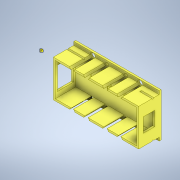
# Autodesk Inventor part: usbHubCaseForTripodClamp
Saved by Autodesk Inventor 2021.2 (Build 252289000, 289)
## iProperties
Created: 2021-02-17
Part Number: usbHubCaseForTripodClamp
Material: PC/ABS Plastic
Document SubType Name: Modeling
Designer: robst
Density: 0.357273 g/cm^3
Appearance: Smooth - Yellow
Author: robst
Autodesk Inventor part; units mm, degrees
ref_plane "YZ Plane" through (0, 0, 0) normal (1, 0, 0) x (0, 1, 0)
ref_plane "XZ Plane" through (0, 0, 0) normal (0, 1, 0) x (-1, 0, 0)
ref_plane "XY Plane" through (0, 0, 0) normal (0, 0, 1) x (1, 0, 0)
sketch "Sketch1" plane through (0, 0, 0) normal (0, 0, 1) x (1, 0, 0)
  line L0 (-57.15, -29.21) -> (57.15, -29.21)
  line L1 (57.15, -29.21) -> (57.15, 29.21)
  line L2 (57.15, 29.21) -> (-57.15, 29.21)
  line L3 (-57.15, 29.21) -> (-57.15, -29.21)
  line L4 (-57.15, -29.21) -> (57.15, 29.21) construction
  line L5 (57.15, -29.21) -> (-57.15, 29.21) construction
  point P0 (0, 0)
  dimension "d0" = 58.42
  dimension "d1" = 114.3
  constraints: 12 end point, 2 midpoint, 2 parallel, 1 horizontal, 1 perpendicular
  measures "d0" distance of L2.end L0.start
  measures "d1" distance of L1.end L2.end
extrude "Extrusion1" add sketch "Sketch1" against normal blind 2.54
sketch "Sketch2" plane through (0, 0, 0) normal (0, 0, 1) x (1, 0, 0)
  line L0 (-57.15, -29.21) -> (-57.15, 29.21) projected
  line L1 (57.15, 29.21) -> (57.15, -29.21) projected
  line L2 (-57.15, 24.765) -> (57.15, 24.765)
  line L3 (57.15, 24.765) -> (57.15, 22.225)
  line L4 (57.15, 22.225) -> (-57.15, 22.225)
  line L5 (-57.15, 22.225) -> (-57.15, 24.765)
  line L6 (-57.15, -24.765) -> (57.15, -24.765)
  line L7 (57.15, -24.765) -> (57.15, -22.225)
  line L8 (57.15, -22.225) -> (-57.15, -22.225)
  line L9 (-57.15, -22.225) -> (-57.15, -24.765)
  point P0 (0, 0)
  point P1 (-57.15, -22.225)
  point P2 (57.15, -24.765)
  dimension "d4" = 2.54
  dimension "d5" = 2.54
  dimension "d6" = 22.225
  dimension "d7" = 22.225
  constraints: 16 end point, 4 parallel, 4 point on line, 2 horizontal, 2 perpendicular
  measures "d4" distance between parallel lines of L4 L2
  measures "d5" distance between parallel lines of L6 L8
  measures "d6" distance from line of L4 point (0, 0)
  measures "d7" distance from line of L8 point (0, 0)
extrude "Extrusion2" add sketch "Sketch2" along normal blind 27.432 contours L0 L8 L1 L6 | L0 L2 L1 L4
sketch "Sketch3" plane through (0, 0, -2.54) normal (0, 0, -1) x (-1, 0, 0)
  line L0 (-12.7, -25.4) -> (12.7, -25.4) construction
  line L1 (12.7, -25.4) -> (12.7, 25.4) construction
  line L2 (12.7, 25.4) -> (-12.7, 25.4) construction
  line L3 (-12.7, 25.4) -> (-12.7, -25.4) construction
  line L4 (-12.7, -25.4) -> (12.7, 25.4) construction
  line L5 (12.7, -25.4) -> (-12.7, 25.4) construction
  point P0 (0, 0)
  dimension "d10" = 25.4
  dimension "d11" = 50.8
  constraints: 12 end point, 4 coincident, 2 midpoint, 2 parallel, 1 horizontal, 1 perpendicular
  measures "d10" distance of L1.end L2.end
  measures "d11" distance of L2.end L0.start
hole "Hole1" at (12.7, 25.4, -2.54) at (-12.7, 25.4, -2.54) at (-12.7, -25.4, -2.54) at (12.7, -25.4, -2.54) direction (0, 0, 1) diameter 3.81 end through all clearance for "Flat Head Machine Screw (82)" size "#6" standard "Ansi Unified Screw Threads"
sketch "Sketch4" plane through (0, 0, 0) normal (0, 0, 1) x (1, 0, 0)
  circle A0 centre (-12.7, 25.4) radius 1.905 projected
  circle A1 centre (-12.7, 25.4) radius 3.81
  circle A2 centre (12.7, 25.4) radius 1.905 projected
  circle A3 centre (12.7, 25.4) radius 3.81
  circle A4 centre (12.7, -25.4) radius 1.905 projected
  circle A5 centre (12.7, -25.4) radius 3.81
  arc A6 (-14.4961, -24.765) -> (-10.9039, -24.765) centre (-12.7, -25.4) ccw projected
  circle A7 centre (-12.7, -25.4) radius 3.81
  point P0 (0, 0)
  dimension "d19" = 7.62
  constraints: 4 centre point, 4 coincident, 3 equal radius
  measures "d19" diameter of A1
extrude "Extrusion3" cut sketch "Sketch4" along normal through all contours A0 | A1 | A2 | A3 | A4 | A5 | A7
sketch "Sketch5" plane through (57.15, -29.21, -2.54) normal (1, 0, 0) x (0, 0, -1)
  line L0 (-29.972, 53.975) -> (-29.972, 51.435) projected
  line L1 (-2.54, 51.435) -> (-2.54, 6.985) projected
  line L2 (-29.972, 51.435) -> (-2.54, 51.435)
  line L3 (-2.54, 51.435) -> (-2.54, 6.985)
  line L4 (-2.54, 6.985) -> (-29.972, 6.985)
  line L5 (-29.972, 6.985) -> (-29.972, 51.435)
  point P0 (-2.54, 29.21)
  constraints: 8 end point, 2 parallel, 1 horizontal, 1 perpendicular
extrude "Extrusion4" add sketch "Sketch5" against normal blind 2.54
sketch "Sketch6" plane through (57.15, -29.21, -2.54) normal (1, 0, 0) x (0, 0, -1)
  line L0 (-2.54, 51.435) -> (-29.972, 51.435) projected
  line L1 (-2.54, 6.985) -> (-2.54, 51.435) projected
  line L2 (-29.972, 6.985) -> (-2.54, 6.985) projected
  line L3 (-29.972, 51.435) -> (-29.972, 53.975) construction
  line L4 (-29.972, 51.435) -> (-2.54, 6.985) construction
  line L5 (-2.54, 51.435) -> (-29.972, 6.985) construction
  line L6 (-23.876, 19.685) -> (-8.636, 19.685)
  line L7 (-8.636, 19.685) -> (-8.636, 38.735)
  line L8 (-8.636, 38.735) -> (-23.876, 38.735)
  line L9 (-23.876, 38.735) -> (-23.876, 19.685)
  line L10 (-23.876, 19.685) -> (-8.636, 38.735) construction
  line L11 (-8.636, 19.685) -> (-23.876, 38.735) construction
  point P0 (-2.54, 29.21)
  point P1 (-16.256, 29.21)
  dimension "d24" = 15.24
  dimension "d25" = 19.05
  constraints: 16 end point, 3 midpoint, 2 parallel, 1 horizontal, 1 perpendicular
  measures "d24" distance of L7.end L8.end
  measures "d25" distance of L6.end L7.end
extrude "Extrusion5" cut sketch "Sketch6" against normal up to surface (2.54 mm away)
sketch "Sketch7" plane through (-57.15, -29.21, -2.54) normal (-1, 0, 0) x (0, 0, 1)
  line L0 (2.54, 51.435) -> (29.972, 51.435) projected
  line L1 (29.972, 6.985) -> (29.972, 51.435) projected
  line L2 (2.54, 6.985) -> (29.972, 6.985) projected
  line L3 (2.54, 51.435) -> (2.54, 6.985) projected
  line L4 (2.54, 6.985) -> (2.54, 51.435) construction
  line L5 (29.972, 6.985) -> (2.54, 6.985) construction
  line L6 (2.54, 51.435) -> (29.972, 6.985) construction
  line L7 (2.54, 51.435) -> (29.972, 51.435) construction
  line L8 (29.972, 51.435) -> (2.54, 6.985) construction
  line L9 (5.461, 13.97) -> (27.051, 13.97)
  line L10 (27.051, 13.97) -> (27.051, 44.45)
  line L11 (27.051, 44.45) -> (5.461, 44.45)
  line L12 (5.461, 44.45) -> (5.461, 13.97)
  line L13 (5.461, 13.97) -> (27.051, 44.45) construction
  line L14 (27.051, 13.97) -> (5.461, 44.45) construction
  point P0 (2.54, 29.21)
  point P1 (16.256, 29.21)
  dimension "d28" = 30.48
  dimension "d29" = 21.59
  constraints: 16 end point, 3 midpoint, 2 parallel, 2 perpendicular
  measures "d28" distance of L11.end L9.start
  measures "d29" distance of L10.end L11.end
extrude "Extrusion6" add sketch "Sketch7" against normal blind 2.54
sketch "Sketch8" plane through (57.15, -29.21, -2.54) normal (1, 0, 0) x (0, 0, -1)
  line L0 (-2.54, 53.975) -> (-29.972, 53.975) projected
  line L1 (-29.972, 53.975) -> (-2.54, 53.975) projected
  line L2 (-12.192, 53.975) -> (-10.922, 52.705)
  line L3 (-10.922, 52.705) -> (-9.652, 53.975)
  line L4 (-9.652, 53.975) -> (-12.192, 53.975)
  line L5 (-29.972, 4.445) -> (-29.972, 53.975) projected
  point P0 (-2.54, 29.21)
  dimension "d32" = 90
  dimension "d33" = 135
  dimension "d34" = 1.27
  dimension "d35" = 19.05
  constraints: 6 end point, 2 point on line, 1 collinear
  measures "d32" angle of L3 L2
  measures "d33" angle of L2 L0
  measures "d34" distance from line of L2.end L0
  measures "d35" distance from line of L2.end L5
extrude "Extrusion7" cut sketch "Sketch8" against normal blind 16.51
mirror "Mirror1" about plane through (0, 0, 0) normal (0, 1, 0) of "Extrusion7"
sketch "Sketch9" plane through (-57.15, -29.21, -2.54) normal (-1, 0, 0) x (0, 0, 1)
  line L0 (9.652, 53.975) -> (10.922, 52.705) projected
  line L1 (10.922, 52.705) -> (12.192, 53.975) projected
  line L2 (2.54, 53.975) -> (29.972, 53.975) projected
  line L3 (12.192, 53.975) -> (10.922, 52.705)
  line L4 (9.652, 53.975) -> (10.922, 52.705) projected
  line L5 (10.922, 52.705) -> (9.652, 53.975)
  line L6 (9.652, 53.975) -> (12.192, 53.975)
  line L7 (2.54, 53.975) -> (29.972, 53.975) projected
  point P0 (2.54, 29.21)
  constraints: 6 end point, 2 collinear
extrude "Extrusion8" cut sketch "Sketch9" against normal blind 27.94
mirror "Mirror2" about plane through (0, 0, 0) normal (0, 1, 0) of "Extrusion8"
sketch "Sketch10" plane through (0, 0, -2.54) normal (0, 0, -1) x (-1, 0, 0)
  line L0 (-31.75, -25.4) -> (31.75, -25.4) construction
  line L1 (31.75, -25.4) -> (31.75, 25.4) construction
  line L2 (31.75, 25.4) -> (-31.75, 25.4) construction
  line L3 (-31.75, 25.4) -> (-31.75, -25.4) construction
  line L4 (-31.75, -25.4) -> (31.75, 25.4) construction
  line L5 (31.75, -25.4) -> (-31.75, 25.4) construction
  point P0 (0, 0)
  dimension "d40" = 63.5
  dimension "d41" = 50.8
  constraints: 12 end point, 4 coincident, 2 midpoint, 2 parallel, 1 horizontal, 1 perpendicular
  measures "d40" distance of L0.start L0.end
  measures "d41" distance of L1.end L0.end
hole "Hole2" at (31.75, 25.4, -2.54) at (-31.75, 25.4, -2.54) at (-31.75, -25.4, -2.54) at (31.75, -25.4, -2.54) direction (0, 0, 1) diameter 6.985 end through all
sketch "Sketch11" plane through (0, 0, 0) normal (0, 0, 1) x (1, 0, 0)
  line L0 (54.61, 9.525) -> (54.61, -9.525) construction
  line L1 (54.61, 0) -> (-54.61, 0) construction
  line L2 (-54.61, 22.225) -> (-54.61, -22.225) construction
  line L3 (-29.5043, -3.81) -> (-30.5171, -3.81)
  line L4 (-30.5171, -3.81) -> (-30.5171, -0.0803)
  line L5 (-30.5171, -0.0803) -> (-34.0245, -0.0803)
  line L6 (-34.0245, -0.0803) -> (-34.0245, -3.81)
  line L7 (-34.0245, -3.81) -> (-35.0372, -3.81)
  line L8 (-35.0372, -3.81) -> (-35.0372, 3.81)
  line L9 (-35.0372, 3.81) -> (-34.0245, 3.81)
  line L10 (-34.0245, 3.81) -> (-34.0245, 0.8213)
  line L11 (-34.0245, 0.8213) -> (-30.5171, 0.8213)
  line L12 (-30.5171, 0.8213) -> (-30.5171, 3.81)
  line L13 (-30.5171, 3.81) -> (-29.5043, 3.81)
  line L14 (-29.5043, 3.81) -> (-29.5043, -3.81)
  spline S0 degree 2 poles (-25.8364, -3.9459) (-26.6638, -3.9459) (-27.8247, -3.6) (-28.3373, -3.353) knots 0 0 0 1 2 2 2
  line L15 (-28.3373, -3.353) -> (-28.3373, -2.081)
  line L16 (-28.3373, -2.081) -> (-28.2632, -2.081)
  spline S1 degree 2 poles (-28.2632, -2.081) (-27.763, -2.5503) (-26.4971, -3.069) (-25.9105, -3.069) knots 0 0 0 1 2 2 2
  spline S2 degree 2 poles (-25.9105, -3.069) (-25.0707, -3.069) (-24.2123, -2.3712) (-24.2123, -1.7969) knots 0 0 0 1 2 2 2
  spline S3 degree 2 poles (-24.2123, -1.7969) (-24.2123, -1.34) (-24.6631, -0.7719) (-25.1509, -0.6299) knots 0 0 0 1 2 2 2
  spline S4 degree 2 poles (-25.1509, -0.6299) (-25.5029, -0.5311) (-26.0895, -0.3952) (-26.528, -0.2841) knots 0 0 0 1 2 2 2
  spline S5 degree 2 poles (-26.528, -0.2841) (-26.9232, -0.1791) (-27.5469, 0.1359) (-27.7877, 0.389) knots 0 0 0 1 2 2 2
  spline S6 degree 2 poles (-27.7877, 0.389) (-28.0223, 0.6422) (-28.2817, 1.3215) (-28.2817, 1.7661) knots 0 0 0 1 2 2 2
  spline S7 degree 2 poles (-28.2817, 1.7661) (-28.2817, 2.6923) (-26.8367, 3.9459) (-25.719, 3.9459) knots 0 0 0 1 2 2 2
  spline S8 degree 2 poles (-25.719, 3.9459) (-25.0768, 3.9459) (-23.9406, 3.6927) (-23.4528, 3.4518) knots 0 0 0 1 2 2 2
  line L17 (-23.4528, 3.4518) -> (-23.4528, 2.2415)
  line L18 (-23.4528, 2.2415) -> (-23.5269, 2.2415)
  spline S9 degree 2 poles (-23.5269, 2.2415) (-23.8912, 2.575) (-25.0274, 3.069) (-25.6511, 3.069) knots 0 0 0 1 2 2 2
  spline S10 degree 2 poles (-25.6511, 3.069) (-26.3551, 3.069) (-27.2258, 2.4083) (-27.2258, 1.871) knots 0 0 0 1 2 2 2
  spline S11 degree 2 poles (-27.2258, 1.871) (-27.2258, 1.3894) (-26.7132, 0.8151) (-26.2316, 0.6854) knots 0 0 0 1 2 2 2
  spline S12 degree 2 poles (-26.2316, 0.6854) (-25.9105, 0.599) (-24.978, 0.3767) (-24.6693, 0.2841) knots 0 0 0 1 2 2 2
  spline S13 degree 2 poles (-24.6693, 0.2841) (-23.8851, 0.0432) (-23.1564, -0.9263) (-23.1564, -1.6364) knots 0 0 0 1 2 2 2
  spline S14 degree 2 poles (-23.1564, -1.6364) (-23.1564, -2.0872) (-23.5207, -2.9517) (-23.848, -3.2542) knots 0 0 0 1 2 2 2
  spline S15 degree 2 poles (-23.848, -3.2542) (-24.2123, -3.5877) (-25.1386, -3.9459) (-25.8364, -3.9459) knots 0 0 0 1 2 2 2
  spline S16 degree 2 poles (-16.9567, -1.4697) (-16.9567, -2.0378) (-17.3889, -2.9084) (-17.7471, -3.1925) knots 0 0 0 1 2 2 2
  spline S17 degree 2 poles (-17.7471, -3.1925) (-18.1793, -3.5259) (-19.1612, -3.81) (-19.9392, -3.81) knots 0 0 0 1 2 2 2
  line L19 (-19.9392, -3.81) -> (-22.1252, -3.81)
  line L20 (-22.1252, -3.81) -> (-22.1252, 3.81)
  line L21 (-22.1252, 3.81) -> (-20.1059, 3.81)
  spline S18 degree 2 poles (-20.1059, 3.81) (-19.2908, 3.81) (-18.4757, 3.705) (-18.1052, 3.5012) knots 0 0 0 1 2 2 2
  spline S19 degree 2 poles (-18.1052, 3.5012) (-17.6915, 3.2851) (-17.3148, 2.575) (-17.3148, 2.0933) knots 0 0 0 1 2 2 2
  spline S20 degree 2 poles (-17.3148, 2.0933) (-17.3148, 1.5561) (-17.8829, 0.704) (-18.3831, 0.4631) knots 0 0 0 1 2 2 2
  line L22 (-18.3831, 0.4631) -> (-18.3831, 0.4261)
  spline S21 degree 2 poles (-18.3831, 0.4261) (-17.7038, 0.2408) (-16.9567, -0.741) (-16.9567, -1.4697) knots 0 0 0 1 2 2 2
  spline S22 degree 2 poles (-18.0126, -1.5129) (-18.0126, -1.0806) (-18.2596, -0.5249) (-18.6301, -0.3273) knots 0 0 0 1 2 2 2
  spline S23 degree 2 poles (-18.6301, -0.3273) (-18.8709, -0.2038) (-19.439, -0.1297) (-19.9639, -0.1297) knots 0 0 0 1 2 2 2
  line L23 (-19.9639, -0.1297) -> (-21.1125, -0.1297)
  line L24 (-21.1125, -0.1297) -> (-21.1125, -2.9455)
  line L25 (-21.1125, -2.9455) -> (-20.2912, -2.9455)
  spline S24 degree 2 poles (-20.2912, -2.9455) (-19.6243, -2.9455) (-18.8586, -2.822) (-18.5622, -2.6244) knots 0 0 0 1 2 2 2
  spline S25 degree 2 poles (-18.5622, -2.6244) (-18.2781, -2.4206) (-18.0126, -1.9143) (-18.0126, -1.5129) knots 0 0 0 1 2 2 2
  spline S26 degree 2 poles (-18.3707, 1.9513) (-18.3707, 2.223) (-18.556, 2.6306) (-18.7598, 2.7479) knots 0 0 0 1 2 2 2
  spline S27 degree 2 poles (-18.7598, 2.7479) (-19.0068, 2.8837) (-19.6058, 2.9455) (-20.143, 2.9455) knots 0 0 0 1 2 2 2
  line L26 (-20.143, 2.9455) -> (-21.1125, 2.9455)
  line L27 (-21.1125, 2.9455) -> (-21.1125, 0.7163)
  line L28 (-21.1125, 0.7163) -> (-19.9639, 0.7163)
  spline S28 degree 2 poles (-19.9639, 0.7163) (-19.4884, 0.7163) (-19.0377, 0.8151) (-18.7968, 0.9695) knots 0 0 0 1 2 2 2
  spline S29 degree 2 poles (-18.7968, 0.9695) (-18.5622, 1.1177) (-18.3707, 1.5932) (-18.3707, 1.9513) knots 0 0 0 1 2 2 2
  line L29 (-7.1445, -3.81) -> (-8.1572, -3.81)
  line L30 (-8.1572, -3.81) -> (-8.1572, -0.0803)
  line L31 (-8.1572, -0.0803) -> (-11.6647, -0.0803)
  line L32 (-11.6647, -0.0803) -> (-11.6647, -3.81)
  line L33 (-11.6647, -3.81) -> (-12.6774, -3.81)
  line L34 (-12.6774, -3.81) -> (-12.6774, 3.81)
  line L35 (-12.6774, 3.81) -> (-11.6647, 3.81)
  line L36 (-11.6647, 3.81) -> (-11.6647, 0.8213)
  line L37 (-11.6647, 0.8213) -> (-8.1572, 0.8213)
  line L38 (-8.1572, 0.8213) -> (-8.1572, 3.81)
  line L39 (-8.1572, 3.81) -> (-7.1445, 3.81)
  line L40 (-7.1445, 3.81) -> (-7.1445, -3.81)
  line L41 (-1.2288, -3.81) -> (-2.1921, -3.81)
  line L42 (-2.1921, -3.81) -> (-2.1921, -3.1801)
  spline S30 degree 2 poles (-2.1921, -3.1801) (-2.6367, -3.5692) (-3.4333, -3.9706) (-3.9273, -3.9706) knots 0 0 0 1 2 2 2
  spline S31 degree 2 poles (-3.9273, -3.9706) (-4.2978, -3.9706) (-4.9586, -3.7235) (-5.1994, -3.458) knots 0 0 0 1 2 2 2
  spline S32 degree 2 poles (-5.1994, -3.458) (-5.4464, -3.1925) (-5.7181, -2.3836) (-5.7181, -1.8031) knots 0 0 0 1 2 2 2
  line L43 (-5.7181, -1.8031) -> (-5.7181, 1.9081)
  line L44 (-5.7181, 1.9081) -> (-4.7548, 1.9081)
  line L45 (-4.7548, 1.9081) -> (-4.7548, -1.3523)
  spline S33 degree 2 poles (-4.7548, -1.3523) (-4.7548, -1.8093) (-4.6869, -2.4083) (-4.5695, -2.6306) knots 0 0 0 1 2 2 2
  spline S34 degree 2 poles (-4.5695, -2.6306) (-4.4522, -2.8529) (-4.0508, -3.0566) (-3.6742, -3.0566) knots 0 0 0 1 2 2 2
  spline S35 degree 2 poles (-3.6742, -3.0566) (-3.3222, -3.0566) (-2.5256, -2.6553) (-2.1921, -2.365) knots 0 0 0 1 2 2 2
  line L46 (-2.1921, -2.365) -> (-2.1921, 1.9081)
  line L47 (-2.1921, 1.9081) -> (-1.2288, 1.9081)
  line L48 (-1.2288, 1.9081) -> (-1.2288, -3.81)
  spline S36 degree 2 poles (4.9586, -0.8583) (4.9586, -2.2601) (3.6, -3.9706) (2.575, -3.9706) knots 0 0 0 1 2 2 2
  spline S37 degree 2 poles (2.575, -3.9706) (2.1119, -3.9706) (1.4511, -3.7421) (1.13, -3.5445) knots 0 0 0 1 2 2 2
  line L49 (1.13, -3.5445) -> (1.0683, -3.81)
  line L50 (1.0683, -3.81) -> (0.1667, -3.81)
  line L51 (0.1667, -3.81) -> (0.1667, 4.1496)
  line L52 (0.1667, 4.1496) -> (1.13, 4.1496)
  line L53 (1.13, 4.1496) -> (1.13, 1.3091)
  spline S38 degree 2 poles (1.13, 1.3091) (1.4944, 1.6364) (2.3403, 2.0686) (2.8776, 2.0686) knots 0 0 0 1 2 2 2
  spline S39 degree 2 poles (2.8776, 2.0686) (3.847, 2.0686) (4.9586, 0.5187) (4.9586, -0.8583) knots 0 0 0 1 2 2 2
  spline S40 degree 2 poles (3.9644, -0.9324) (3.9644, 0.0926) (3.3407, 1.1547) (2.6491, 1.1547) knots 0 0 0 1 2 2 2
  spline S41 degree 2 poles (2.6491, 1.1547) (2.2601, 1.1547) (1.4573, 0.7842) (1.13, 0.5002) knots 0 0 0 1 2 2 2
  line L54 (1.13, 0.5002) -> (1.13, -2.7788)
  spline S42 degree 2 poles (1.13, -2.7788) (1.4944, -2.9578) (2.0563, -3.106) (2.3897, -3.106) knots 0 0 0 1 2 2 2
  spline S43 degree 2 poles (2.3897, -3.106) (3.1246, -3.106) (3.9644, -2.0625) (3.9644, -0.9324) knots 0 0 0 1 2 2 2
  spline S44 degree 2 poles (14.1223, 1.5129) (14.1223, 1.0189) (13.7703, 0.1297) (13.4554, -0.1791) knots 0 0 0 1 2 2 2
  spline S45 degree 2 poles (13.4554, -0.1791) (13.0602, -0.5681) (11.9919, -0.9695) (11.1768, -0.9695) knots 0 0 0 1 2 2 2
  line L55 (11.1768, -0.9695) -> (10.3185, -0.9695)
  line L56 (10.3185, -0.9695) -> (10.3185, -3.81)
  line L57 (10.3185, -3.81) -> (9.3058, -3.81)
  line L58 (9.3058, -3.81) -> (9.3058, 3.81)
  line L59 (9.3058, 3.81) -> (11.22, 3.81)
  spline S46 degree 2 poles (11.22, 3.81) (11.8993, 3.81) (12.8503, 3.5877) (13.2146, 3.3345) knots 0 0 0 1 2 2 2
  spline S47 degree 2 poles (13.2146, 3.3345) (13.6407, 3.0443) (14.1223, 2.1489) (14.1223, 1.5129) knots 0 0 0 1 2 2 2
  spline S48 degree 2 poles (13.0664, 1.482) (13.0664, 1.8772) (12.7947, 2.4577) (12.5168, 2.6429) knots 0 0 0 1 2 2 2
  spline S49 degree 2 poles (12.5168, 2.6429) (12.276, 2.8035) (11.6338, 2.9331) (11.1583, 2.9331) knots 0 0 0 1 2 2 2
  line L60 (11.1583, 2.9331) -> (10.3185, 2.9331)
  line L61 (10.3185, 2.9331) -> (10.3185, -0.105)
  line L62 (10.3185, -0.105) -> (11.0101, -0.105)
  spline S50 degree 2 poles (11.0101, -0.105) (11.6276, -0.105) (12.3871, 0.0926) (12.6341, 0.352) knots 0 0 0 1 2 2 2
  spline S51 degree 2 poles (12.6341, 0.352) (12.8626, 0.5805) (13.0664, 1.1177) (13.0664, 1.482) knots 0 0 0 1 2 2 2
  line L63 (20.6123, 3.81) -> (17.9879, -3.81)
  line L64 (17.9879, -3.81) -> (16.8949, -3.81)
  line L65 (16.8949, -3.81) -> (14.2705, 3.81)
  line L66 (14.2705, 3.81) -> (15.3573, 3.81)
  line L67 (15.3573, 3.81) -> (17.4692, -2.5194)
  line L68 (17.4692, -2.5194) -> (19.5811, 3.81)
  line L69 (19.5811, 3.81) -> (20.6123, 3.81)
  line L70 (24.0024, -0.9386) -> (21.1186, -0.9386)
  line L71 (21.1186, -0.9386) -> (21.1186, -0.0123)
  line L72 (21.1186, -0.0123) -> (24.0024, -0.0123)
  line L73 (24.0024, -0.0123) -> (24.0024, -0.9386)
  spline S52 degree 2 poles (29.7575, 0) (29.7575, -2.0501) (28.5657, -3.9706) (27.3246, -3.9706) knots 0 0 0 1 2 2 2
  spline S53 degree 2 poles (27.3246, -3.9706) (26.0648, -3.9706) (24.8854, -2.0131) (24.8854, -0.0062) knots 0 0 0 1 2 2 2
  spline S54 degree 2 poles (24.8854, -0.0062) (24.8854, 2.0563) (26.0772, 3.9644) (27.3246, 3.9644) knots 0 0 0 1 2 2 2
  spline S55 degree 2 poles (27.3246, 3.9644) (28.5781, 3.9644) (29.7575, 1.9884) (29.7575, 0) knots 0 0 0 1 2 2 2
  spline S56 degree 2 poles (28.4484, -2.3218) (28.5966, -1.9451) (28.7201, -0.7842) (28.7201, 0) knots 0 0 0 1 2 2 2
  spline S57 degree 2 poles (28.7201, 0) (28.7201, 0.7842) (28.5966, 1.939) (28.4422, 2.328) knots 0 0 0 1 2 2 2
  spline S58 degree 2 poles (28.4422, 2.328) (28.2879, 2.717) (27.7506, 3.1184) (27.3246, 3.1184) knots 0 0 0 1 2 2 2
  spline S59 degree 2 poles (27.3246, 3.1184) (26.8985, 3.1184) (26.3489, 2.717) (26.1883, 2.3156) knots 0 0 0 1 2 2 2
  spline S60 degree 2 poles (26.1883, 2.3156) (26.034, 1.9266) (25.9228, 0.741) (25.9228, -0.0062) knots 0 0 0 1 2 2 2
  spline S61 degree 2 poles (25.9228, -0.0062) (25.9228, -0.8089) (26.0216, -1.8834) (26.1822, -2.3033) knots 0 0 0 1 2 2 2
  spline S62 degree 2 poles (26.1822, -2.3033) (26.3304, -2.6985) (26.88, -3.1246) (27.3246, -3.1246) knots 0 0 0 1 2 2 2
  spline S63 degree 2 poles (27.3246, -3.1246) (27.7445, -3.1246) (28.294, -2.7232) (28.4484, -2.3218) knots 0 0 0 1 2 2 2
  line L74 (35.4324, -3.81) -> (30.7332, -3.81)
  line L75 (30.7332, -3.81) -> (30.7332, -2.7294)
  spline S64 degree 2 poles (30.7332, -2.7294) (31.2395, -2.2539) (32.1411, -1.3709) (32.5733, -0.8954) knots 0 0 0 1 2 2 2
  spline S65 degree 2 poles (32.5733, -0.8954) (33.444, 0.0618) (34.08, 1.2103) (34.08, 1.8216) knots 0 0 0 1 2 2 2
  spline S66 degree 2 poles (34.08, 1.8216) (34.08, 2.1427) (33.8824, 2.6244) (33.7034, 2.7788) knots 0 0 0 1 2 2 2
  spline S67 degree 2 poles (33.7034, 2.7788) (33.5243, 2.9331) (33.055, 3.0875) (32.7709, 3.0875) knots 0 0 0 1 2 2 2
  spline S68 degree 2 poles (32.7709, 3.0875) (32.4992, 3.0875) (31.9435, 2.9517) (31.6903, 2.8467) knots 0 0 0 1 2 2 2
  spline S69 degree 2 poles (31.6903, 2.8467) (31.4742, 2.7602) (31.0728, 2.5132) (30.9493, 2.4268) knots 0 0 0 1 2 2 2
  line L76 (30.9493, 2.4268) -> (30.8937, 2.4268)
  line L77 (30.8937, 2.4268) -> (30.8937, 3.5136)
  spline S70 degree 2 poles (30.8937, 3.5136) (31.2087, 3.668) (32.3387, 3.9706) (32.845, 3.9706) knots 0 0 0 1 2 2 2
  spline S71 degree 2 poles (32.845, 3.9706) (33.9133, 3.9706) (35.1175, 2.8405) (35.1175, 1.8772) knots 0 0 0 1 2 2 2
  spline S72 degree 2 poles (35.1175, 1.8772) (35.1175, 1.4264) (34.9075, 0.6731) (34.7223, 0.352) knots 0 0 0 1 2 2 2
  spline S73 degree 2 poles (34.7223, 0.352) (34.537, 0.0185) (33.9998, -0.636) (33.7034, -0.951) knots 0 0 0 1 2 2 2
  spline S74 degree 2 poles (33.7034, -0.951) (33.2217, -1.4758) (32.0423, -2.5997) (31.6903, -2.927) knots 0 0 0 1 2 2 2
  line L78 (31.6903, -2.927) -> (35.4324, -2.927)
  line L79 (35.4324, -2.927) -> (35.4324, -3.81)
  point P0 (0, 0)
  constraints: 2 end point, 2 midpoint, 1 horizontal
extrude "Extrusion9" cut sketch "Sketch11" against normal blind 1.27
equation "\"d0\" = usbHolderWidth"
equation "\"d1\" = usbHolderLength"
equation "\"d2\" = usbHolderWallThickness"
equation "\"d4\" = usbHolderWallThickness"
equation "\"d5\" = usbHolderWallThickness"
equation "\"d6\" = 0.5 * usbHubWidth"
equation "\"d7\" = 0.5 * usbHubWidth"
equation "\"d8\" = usbHubDepth"
equation "\"d10\" = holePatternLength"
equation "\"d11\" = holePatternWidth"
equation "\"d22\" = usbHolderWallThickness"
equation "\"d26\" = usbHolderWallThickness"
equation "\"d30\" = usbHolderWallThickness"
equation "\"usbHolderWallThickness\" = 2.54"
equation "\"usbHubWidth\" = 44.45"
equation "\"usbHubDepth\" = 27.432"
equation "\"usbHubLength\" = 109.22"
equation "\"usbHolderWidth\" = 58.42"
equation "\"usbHolderLength\" = usbHubLength + 2 * usbHolderWallThickness"
equation "\"holePatternLength\" = 25.4"
equation "\"holePatternWidth\" = 50.8"
body "Solid1"
